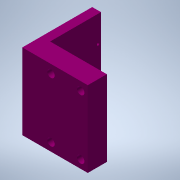
# Autodesk Inventor part: beam steering subassy mounting bracket
Saved by Autodesk Inventor 2022 (Build 260153000, 153)
## iProperties
Created: 2011-09-10
Part Number: beam steering subassy mounting bracket
Document SubType Name: Modeling
Designer: betzige
Density: 1 g/cm^3
Material: Generic
Appearance: Magenta Dark
Author: betzige
Autodesk Inventor part; units mm, degrees
ref_plane "YZ Plane" through (0, 0, 0) normal (1, 0, 0) x (0, 1, 0)
ref_plane "XZ Plane" through (0, 0, 0) normal (0, 1, 0) x (-1, 0, 0)
ref_plane "XY Plane" through (0, 0, 0) normal (0, 0, 1) x (1, 0, 0)
sketch "Sketch1" plane through (0, 0, 0) normal (0, 0, 1) x (1, 0, 0)
  line L0 (0, 0) -> (7.5, 0)
  line L1 (7.5, 13) -> (7.5, 56.5)
  line L2 (7.5, 56.5) -> (0, 56.5)
  line L3 (0, 56.5) -> (0, 0)
  line L4 (0, 0) -> (56, 0)
  line L5 (56, 0) -> (56, 13)
  line L6 (56, 13) -> (7.5, 13)
  line L7 (0, 13) -> (0, 0)
  dimension "d0" = 13
  dimension "d1" = 56
  dimension "d2" = 56.5
  dimension "d3" = 7.5
  constraints: 16 end point, 4 parallel, 2 horizontal, 2 perpendicular
  measures "d0" distance between parallel lines of L4 L6
  measures "d1" distance of L0.start L4.end
  measures "d2" distance of L2.end L0.start
  measures "d3" distance of L1.end L2.end
extrude "Extrusion1" add sketch "Sketch1" along normal mid plane 65
sketch "Sketch2" plane through (7.5, 13, 32.5) normal (0, 1, 0) x (1, 0, 0)
  line L0 (0, 0) -> (48.5, 0) projected
  line L1 (48.5, 0) -> (48.5, 65) projected
  line L2 (48.5, 65) -> (0, 65) projected
  line L3 (0, 0) -> (0, 65) projected
  line L4 (42.414, 25.5) -> (42.414, 39.5)
  line L5 (49.414, 32.5) -> (35.414, 32.5)
  point P0 (-7.5, 32.5)
  point P1 (17.014, 57.9)
  point P2 (17.014, 7.1)
  point P3 (42.414, 57.9)
  point P4 (42.414, 7.1)
  dimension "d6" = 25.4
  dimension "d7" = 25.4
  dimension "d8" = 25.4
  dimension "d9" = 25.4
  dimension "d10" = 25.4
  dimension "d11" = 25.4
  dimension "d35" = 25.4
  constraints: 4 end point, 1 horizontal, 1 vertical, 4 other
  measures "d6" distance from line of L4 point (17.014, 57.9)
  measures "d7" distance from line of L5 point (17.014, 57.9)
  measures "d8" distance from line of L5 point (17.014, 7.1)
  measures "d9" distance from line of L4 point (17.014, 7.1)
  measures "d10" distance of point (17.014, 57.9) point (42.414, 57.9)
  measures "d11" distance from line of L5 point (42.414, 57.9)
  measures "d35" distance of point (17.014, 7.1) point (42.414, 7.1)
hole "Hole1" at (24.514, 13, -25.4) at (24.514, 13, 25.4) at (49.914, 13, -25.4) at (49.914, 13, 25.4) direction (0, -1, 0) diameter 6.35 end through all counterbore diameter 10 counterbore depth 6.5
sketch "Sketch3" plane through (7.5, 13, 32.5) normal (0, 1, 0) x (1, 0, 0)
  circle A0 centre (24.9141, 42.5) radius 2.032 projected
  circle A1 centre (24.9141, 22.5) radius 2.032 projected
  circle A2 centre (44.914, 22.5) radius 1.143 projected
  circle A3 centre (44.914, 42.5) radius 1.143 projected
  point P0 (-7.5, 32.5)
hole "Hole2" at (52.414, 13, -10) at (52.414, 13, 10) at (32.4141, 13, 10) at (32.4141, 13, -10) direction (0, -1, 0) diameter 1.694 depth 4 tip angle 118 thread size "2-56 UNC" class "2B" standard "ANSI Unified Screw Threads"
sketch "Sketch4" plane through (0, 0, 32.5) normal (-1, 0, 0) x (0, 0, 1)
  line L0 (0, 56.5) -> (0, 13) projected
  line L1 (0, 13) -> (-65, 13) projected
  line L2 (-65, 13) -> (-65, 56.5) projected
  line L3 (0, 56.5) -> (-65, 56.5) projected
  circle A0 centre (-42.5044, 54.0403) radius 0.889 projected
  circle A1 centre (-22.5044, 34.0403) radius 0.889 projected
  circle A2 centre (-22.5044, 54.0403) radius 1.0922 projected
  line L4 (-45.0044, 32.0483) -> (-45.0044, 31.5403) projected
  line L5 (-45.0044, 31.5403) -> (-20.0044, 31.5403) projected
  line L6 (-20.0044, 31.5403) -> (-20.0044, 56.5403) projected
  line L7 (-20.0044, 56.5403) -> (-45.0044, 56.5403) projected
  line L8 (-45.0044, 56.5403) -> (-45.0044, 56.0323) projected
  line L9 (-45.0044, 56.0323) -> (-45.3092, 56.0323) projected
  line L10 (-45.3092, 32.0483) -> (-45.3092, 56.0323) projected
  line L11 (-45.0044, 32.0483) -> (-45.3092, 32.0483) projected
  circle A3 centre (-42.5044, 34.0403) radius 0.889 projected
  circle A4 centre (-22.5044, 34.0403) radius 0.889 projected
  circle A5 centre (-42.5044, 54.0403) radius 0.889 projected
  circle A6 centre (-22.5044, 54.0403) radius 0.889 projected
  circle A7 centre (-38.8544, 37.6903) radius 1.7272 projected
  circle A8 centre (-26.1544, 37.6903) radius 1.7272 projected
  circle A9 centre (-38.8544, 50.3903) radius 1.7272 projected
  circle A10 centre (-26.1544, 50.3903) radius 1.7272 projected
  circle A11 centre (-32.5044, 44.0403) radius 1.7272 projected
  point P0 (-32.5, 0)
hole "Hole3" at (0, 54.0403, -10.0044) at (0, 54.0403, 9.9956) at (0, 34.0403, 9.9956) at (0, 34.0403, -10.0044) direction (1, 0, 0) diameter 2.1844 end through all counterbore diameter 4 counterbore depth 3
sketch "Sketch5" plane through (7.5, 13, 32.5) normal (1, 0, 0) x (0, 0, -1)
  line L0 (0, 0) -> (65, 0) projected
  line L1 (45.3092, 19.0483) -> (45.3092, 43.0323) projected
  line L2 (65, 43.5) -> (45.3092, 43.5)
  line L3 (45.3092, 43.5) -> (45.3092, 0)
  line L4 (45.3092, 0) -> (65, 0)
  line L5 (65, 0) -> (65, 43.5)
  point P0 (32.5, -13)
  constraints: 8 end point, 2 parallel, 1 horizontal, 1 perpendicular, 1 point on line
extrude "Extrusion2" cut sketch "Sketch5" against normal blind 10
sketch "Sketch6" plane through (0, 0, 32.5) normal (0, -1, 0) x (1, 0, 0)
  circle A0 centre (49.914, -7.1) radius 3.175 projected
  circle A1 centre (49.914, -57.9) radius 3.175 projected
  circle A2 centre (24.514, -7.1) radius 3.175 projected
  circle A3 centre (24.514, -57.9) radius 3.175 projected
  line L0 (56, 0) -> (0, 0) projected
  line L1 (0, -65) -> (0, 0) projected
  line L2 (0, -65) -> (56, -65) projected
  line L3 (56, 0) -> (56, -65) projected
  point P0 (0, -32.5)
extrude "Extrusion3" add sketch "Sketch6" along normal blind 3.3198
body "Solid1"
